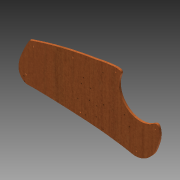
# Autodesk Inventor part: mountingBase02
Saved by Autodesk Inventor 2013 (Build 170138000, 138)
## iProperties
Created: 2014-04-26
Part Number: mountingBase02
Material: Wood (Cherry)
Document SubType Name: Modeling
Designer: Nano
Density: 0.5 g/cm^3
Mass: 26.2829 g
Surface Area: 352.098 cm^2
Volume: 52.5659 cm^3
Author: Nano
Autodesk Inventor part; units mm, degrees
ref_plane "YZ Plane" through (0, 0, 0) normal (1, 0, 0) x (0, 1, 0)
ref_plane "XZ Plane" through (0, 0, 0) normal (0, 1, 0) x (-1, 0, 0)
ref_plane "XY Plane" through (0, 0, 0) normal (0, 0, 1) x (1, 0, 0)
sketch "Sketch1" plane through (0, 0, 0) normal (0, 0, 1) x (1, 0, 0)
  circle A0 centre (22.4774, 26.9707) radius 1.5875 construction
  circle A1 centre (125.529, -53.0458) radius 1.5875 construction
  circle A2 centre (-41.4513, 10.4793) radius 1.5875 construction
  circle A3 centre (-53.6193, -34.8433) radius 1.5875 construction
  circle A4 centre (92.0523, 41.3343) radius 1.5875 construction
  circle A5 centre (156.384, -7.2553) radius 1.5875 construction
  circle A6 centre (34.8781, -43.685) radius 1.5875 construction
  spline S0 degree 4 poles (-47.5552, 16.3255) (-56.6287, 2.113) (-58.2297, -5.7038) (-64.6, -14.5986) (-66.079, -30.6977) (-65.3382, -34.7532) (-63.7847, -39.1481) (-60.7246, -43.61) (-57.2762, -46.3652) (-54.2619, -47.5537) (-52.1718, -47.8438) knots 0 0 0 0 0 0.364781 0.475074 0.575005 0.66288 0.74023 0.816344 1 1 1 1 1
  spline S1 degree 2 poles (58.7626, 42.8458) (4.2199, 34.129) (-47.5552, 16.3255) knots 0 0 0 1 1 1
  spline S2 degree 4 poles (99.6942, 39.5117) (100.5318, 41.9331) (102.2763, 45.9453) (95.6139, 49.3748) (84.6716, 47.1993) (75.6927, 46.6375) (58.7626, 42.8458) knots 0 0 0 0 0 0.302268 0.437081 1 1 1 1 1
  arc A7 (99.6942, 39.5117) -> (153.3806, -0.867) centre (132.2899, 26.9707) ccw
  spline S3 degree 4 poles (-52.1718, -47.8438) (-36.534, -47.2807) (-10.4713, -48.0839) (24.7022, -49.5616) (67.224, -52.2682) (90.8103, -55.4618) (116.0621, -59.11) (123.6332, -61.9611) (134.6518, -59.1205) (140.3655, -56.3824) (147.0585, -51.5689) (152.6758, -44.8659) (156.5759, -39.5192) (161.1474, -26.3914) (163.713, -18.7298) (163.8259, -8.1408) (162.8831, -4.127) (161.1298, 0.7169) (158.3923, 2.1696) (155.7665, 0.7307) (153.3806, -0.867) knots 0 0 0 0 0 0.199945 0.282515 0.361523 0.429863 0.488286 0.53653 0.578018 0.619244 0.659617 0.703918 0.750179 0.797252 0.841669 0.879198 0.910002 0.934908 1 1 1 1 1
  circle A8 centre (-41.4513, 10.4793) radius 1.016
  circle A9 centre (22.4774, 26.9707) radius 1.016
  circle A10 centre (92.0523, 41.3343) radius 1.016
  circle A11 centre (156.384, -7.1763) radius 1.016
  circle A12 centre (125.529, -53.0458) radius 1.016
  circle A13 centre (34.8781, -43.685) radius 1.016
  circle A14 centre (-53.6193, -34.8433) radius 1.016
  point P0 (-58.1503, -3.4556)
  point P1 (-61.848, -12.1317)
  point P2 (-64.9126, -22.073)
  point P3 (-65.6993, -31.3231)
  point P4 (-64.9927, -35.4369)
  point P5 (-63.5229, -39.1631)
  point P6 (-61.3341, -42.4183)
  point P7 (-58.5466, -45.0642)
  point P8 (-55.3853, -46.9262)
  point P9 (4.7943, 31.828)
  point P10 (100.8602, 43.7772)
  point P11 (100.1647, 46.1477)
  point P12 (97.4566, 47.5413)
  point P13 (92.3454, 47.9534)
  point P14 (84.3053, 47.3258)
  point P15 (-26.9279, -47.7688)
  point P16 (3.8331, -48.7884)
  point P17 (37.2041, -50.4527)
  point P18 (68.9139, -52.8419)
  point P19 (96.8666, -56.3799)
  point P20 (117.5981, -59.9718)
  point P21 (125.9835, -60.7611)
  point P22 (134.5495, -58.8078)
  point P23 (140.4841, -56.0058)
  point P24 (146.5962, -51.4173)
  point P25 (152.0147, -45.51)
  point P26 (156.0745, -39.2339)
  point P27 (160.8814, -27.0309)
  point P28 (163.3992, -16.4807)
  point P29 (163.3984, -7.1763)
  point P30 (162.4893, -3.2093)
  point P31 (161.1529, -0.4019)
  point P32 (159.493, 1.023)
  point P33 (157.3678, 1.1626)
  dimension "d2" = 2.032
  dimension "d3" = 2.032
  dimension "d4" = 2.032
  dimension "d5" = 2.032
  dimension "d6" = 2.032
  dimension "d7" = 2.032
  dimension "d8" = 2.032
  constraints: 15 centre point, 2 point on circle, 42 other
  measures "d2" diameter of A8
  measures "d3" diameter of A9
  measures "d4" diameter of A10
  measures "d5" diameter of A11
  measures "d6" diameter of A12
  measures "d7" diameter of A13
  measures "d8" diameter of A14
extrude "Extrusion1" add sketch "Sketch1" against normal blind 3.175
body "Solid1"
